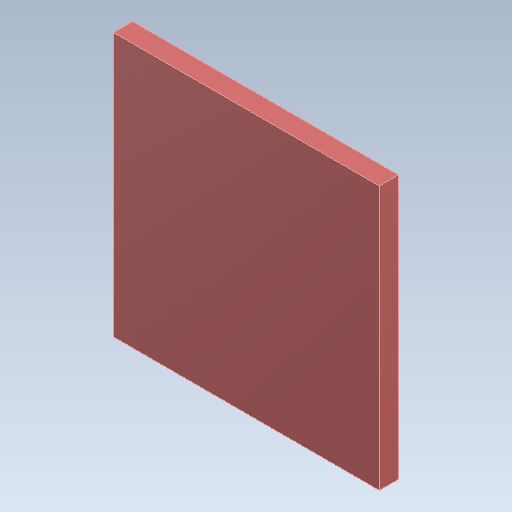
# Autodesk Inventor part: TM4C123GH6PM
Saved by Autodesk Inventor 2021 (Build 250183000, 183)
## iProperties
Created: 2020-11-03
Part Number: TM4C123GH6PM
Material: Generic
Document SubType Name: Modeling
Designer: faiya
Density: 1 g/cm^3
Appearance: SQFP-S-10X10-64, TM4C123GH6PM
Author: faiya
Autodesk Inventor part; units mm, degrees
ref_plane "YZ Plane" through (0, 0, 0) normal (1, 0, 0) x (0, 1, 0)
ref_plane "XZ Plane" through (0, 0, 0) normal (0, 1, 0) x (-1, 0, 0)
ref_plane "XY Plane" through (0, 0, 0) normal (0, 0, 1) x (1, 0, 0)
sketch "SQFP-S-10X10-64, TM4C123GH6PM_44" plane through (0, 0, 0) normal (0, 0, 1) x (1, 0, 0)
  line L0 (-6.9999, 6.9999) -> (6.9999, 6.9999)
  line L1 (6.9999, 6.9999) -> (6.9999, -6.9)
  line L2 (6.9999, -6.9) -> (-6.9999, -6.9)
  line L3 (-6.9999, -6.9) -> (-6.9999, 6.9999)
  constraints: 8 end point
extrude "Extrusion1" add sketch "SQFP-S-10X10-64, TM4C123GH6PM_44" along normal blind 1
body "Solid1"
